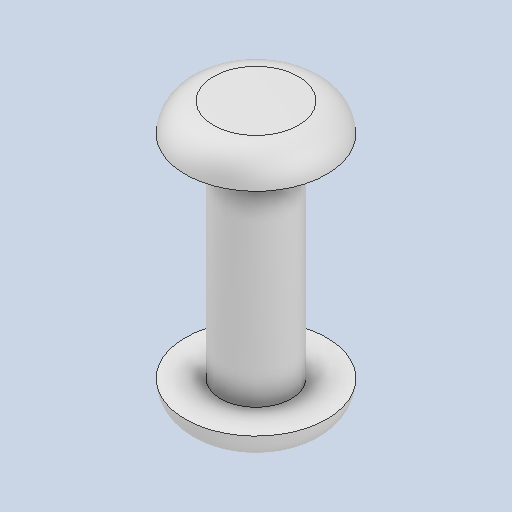
# Autodesk Inventor part: nit_skrecany
Saved by Autodesk Inventor 2024.2 (Build 282272000, 272)
## iProperties
Created: 2024-01-15
Part Number: nit_skrecany
Material: Aluminium
Document SubType Name: Modeling
Designer: Konrad
Density: 2.7 g/cm^3
Appearance: Satynowy
Author: Konrad
Autodesk Inventor part; units mm, degrees
ref_plane "YZ Plane" through (0, 0, 0) normal (1, 0, 0) x (0, 1, 0)
ref_plane "XZ Plane" through (0, 0, 0) normal (0, 1, 0) x (-1, 0, 0)
ref_plane "XY Plane" through (0, 0, 0) normal (0, 0, 1) x (1, 0, 0)
sketch "Szkic1" plane through (0, 0, 0) normal (0, 1, 0) x (-1, 0, 0)
  circle A0 centre (0, 0) radius 2.5
  circle A1 centre (0, 0) radius 5
  dimension "d0" = 5
  dimension "d1" = 10
  constraints: 2 centre point, 2 coincident
  measures "d0" diameter of A0
  measures "d1" diameter of A1
extrude "Wyciągnięcie proste1" add sketch "Szkic1" against normal blind 2 contours A0 | A1
extrude "Wyciągnięcie proste2" add sketch "Szkic1" along normal blind 17 contours A0 | A1
extrude "Wyciągnięcie proste3" cut sketch "Szkic1" along normal blind 15
fillet "Zaokrąglenie1" radius 2 2 edges at (5, 17, 0) (5, -2, 0)
